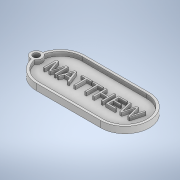
# Autodesk Inventor part: name_tag
Saved by Autodesk Inventor 2020 (Build 240168000, 168)
## iProperties
Created: 2022-11-14
Part Number: name_tag
Material: Generic
Document SubType Name: Modeling
Designer: Matthew Ng
Density: 1 g/cm^3
Appearance: Default
Author: Matthew Ng
Autodesk Inventor part; units mm, degrees
ref_plane "YZ Plane" through (0, 0, 0) normal (1, 0, 0) x (0, 1, 0)
ref_plane "XZ Plane" through (0, 0, 0) normal (0, 1, 0) x (-1, 0, 0)
ref_plane "XY Plane" through (0, 0, 0) normal (0, 0, 1) x (1, 0, 0)
sketch "Sketch1" plane through (0, 0, 0) normal (0, 1, 0) x (-1, 0, 0)
  line L0 (-15, 0) -> (-55, 0)
  line L1 (-55, -30) -> (-15, -30)
  arc A0 (-55, 0) -> (-55, -30) centre (-55, -15) ccw
  line L2 (-15, -1.5) -> (-55, -1.5)
  line L3 (-55, -28.5) -> (-15, -28.5)
  arc A1 (-55, -1.5) -> (-55, -28.5) centre (-55, -15) ccw
  circle A2 centre (0, -15) radius 2
  circle A3 centre (0, -15) radius 3.5
  arc A4 (-15, -28.5) -> (-1.8333, -17.9814) centre (-15, -15) ccw
  arc A5 (-1.8333, -12.0186) -> (-15, -1.5) centre (-15, -15) ccw
  arc A6 (-15, -30) -> (-0.4083, -18.4761) centre (-15, -15) ccw
  arc A7 (-0.4083, -11.5239) -> (-15, 0) centre (-15, -15) ccw
  point P0 (0, 0)
  point P1 (-35, -15)
  dimension "d2" = 30
  dimension "d4" = 27
  dimension "d8" = 7
  dimension "d9" = 4
  constraints: 16 point on circle, 8 centre point, 8 end point, 4 tangent, 2 parallel, 1 coincident, 1 horizontal
  measures "d2" distance between parallel lines of L0 L1
  measures "d4" diameter of A1
  measures "d8" diameter of A3
  measures "d9" diameter of A2
extrude "Extrusion1" add sketch "Sketch1" along normal blind 1.5 contours A3 A4 L3 A1 L2 A5
extrude "Extrusion2" add sketch "Sketch1" along normal blind 4 contours A7 A3 A5 L2 A1 L3 A4 A6 L1 A0 L0 | A3
sketch "Sketch2" plane through (0, 1.5, 0) normal (0, 1, 0) x (1, 0, 0)
  line L0 (7.3671, 19.168) -> (39.5227, 19.168) construction
  line L1 (39.5227, 19.168) -> (39.5227, 12.4254) construction
  line L2 (39.5227, 12.4254) -> (7.3671, 12.4254) construction
  line L3 (7.3671, 12.4254) -> (7.3671, 19.168) construction
  line L4 (8.1964, 11.168) -> (8.1964, 19.168)
  line L5 (8.1964, 19.168) -> (9.7878, 19.168)
  line L6 (9.7878, 19.168) -> (11.6842, 13.5034)
  spline S0 degree 2 poles (11.6842, 13.5034) (11.9464, 12.7107) (12.0683, 12.3204) knots 0 0 0 1 1 1
  spline S1 degree 2 poles (12.0683, 12.3204) (12.2025, 12.7534) (12.4951, 13.6009) knots 0 0 0 1 1 1
  line L7 (12.4951, 13.6009) -> (14.4159, 19.168)
  line L8 (14.4159, 19.168) -> (15.8366, 19.168)
  line L9 (15.8366, 19.168) -> (15.8366, 11.168)
  line L10 (15.8366, 11.168) -> (14.8183, 11.168)
  line L11 (14.8183, 11.168) -> (14.8183, 17.8631)
  line L12 (14.8183, 17.8631) -> (12.4829, 11.168)
  line L13 (12.4829, 11.168) -> (11.5317, 11.168)
  line L14 (11.5317, 11.168) -> (9.2147, 17.979)
  line L15 (9.2147, 17.979) -> (9.2147, 11.168)
  line L16 (9.2147, 11.168) -> (8.1964, 11.168)
  line L17 (16.6659, 11.168) -> (19.739, 19.168)
  line L18 (19.739, 19.168) -> (20.8854, 19.168)
  line L19 (20.8854, 19.168) -> (24.1537, 11.168)
  line L20 (24.1537, 11.168) -> (22.9464, 11.168)
  line L21 (22.9464, 11.168) -> (22.0195, 13.5887)
  line L22 (22.0195, 13.5887) -> (18.6659, 13.5887)
  line L23 (18.6659, 13.5887) -> (17.7878, 11.168)
  line L24 (17.7878, 11.168) -> (16.6659, 11.168)
  line L25 (18.9708, 14.4485) -> (21.6903, 14.4485)
  line L26 (21.6903, 14.4485) -> (20.8488, 16.668)
  spline S2 degree 2 poles (20.8488, 16.668) (20.4708, 17.6802) (20.2878, 18.3265) knots 0 0 0 1 1 1
  spline S3 degree 2 poles (20.2878, 18.3265) (20.1293, 17.5582) (19.8549, 16.796) knots 0 0 0 1 1 1
  line L27 (19.8549, 16.796) -> (18.9708, 14.4485)
  line L28 (27.0317, 11.168) -> (27.0317, 18.2229)
  line L29 (27.0317, 18.2229) -> (24.3976, 18.2229)
  line L30 (24.3976, 18.2229) -> (24.3976, 19.168)
  line L31 (24.3976, 19.168) -> (30.739, 19.168)
  line L32 (30.739, 19.168) -> (30.739, 18.2229)
  line L33 (30.739, 18.2229) -> (28.0927, 18.2229)
  line L34 (28.0927, 18.2229) -> (28.0927, 11.168)
  line L35 (28.0927, 11.168) -> (27.0317, 11.168)
  line L36 (33.861, 11.168) -> (33.861, 18.2229)
  line L37 (33.861, 18.2229) -> (31.2269, 18.2229)
  line L38 (31.2269, 18.2229) -> (31.2269, 19.168)
  line L39 (31.2269, 19.168) -> (37.5683, 19.168)
  line L40 (37.5683, 19.168) -> (37.5683, 18.2229)
  line L41 (37.5683, 18.2229) -> (34.922, 18.2229)
  line L42 (34.922, 18.2229) -> (34.922, 11.168)
  line L43 (34.922, 11.168) -> (33.861, 11.168)
  line L44 (38.6964, 11.168) -> (38.6964, 19.168)
  line L45 (38.6964, 19.168) -> (39.7573, 19.168)
  line L46 (39.7573, 19.168) -> (39.7573, 15.8814)
  line L47 (39.7573, 15.8814) -> (43.9037, 15.8814)
  line L48 (43.9037, 15.8814) -> (43.9037, 19.168)
  line L49 (43.9037, 19.168) -> (44.9647, 19.168)
  line L50 (44.9647, 19.168) -> (44.9647, 11.168)
  line L51 (44.9647, 11.168) -> (43.9037, 11.168)
  line L52 (43.9037, 11.168) -> (43.9037, 14.9363)
  line L53 (43.9037, 14.9363) -> (39.7573, 14.9363)
  line L54 (39.7573, 14.9363) -> (39.7573, 11.168)
  line L55 (39.7573, 11.168) -> (38.6964, 11.168)
  line L56 (46.7512, 11.168) -> (46.7512, 19.168)
  line L57 (46.7512, 19.168) -> (52.5439, 19.168)
  line L58 (52.5439, 19.168) -> (52.5439, 18.2229)
  line L59 (52.5439, 18.2229) -> (47.8122, 18.2229)
  line L60 (47.8122, 18.2229) -> (47.8122, 15.7778)
  line L61 (47.8122, 15.7778) -> (52.2451, 15.7778)
  line L62 (52.2451, 15.7778) -> (52.2451, 14.8326)
  line L63 (52.2451, 14.8326) -> (47.8122, 14.8326)
  line L64 (47.8122, 14.8326) -> (47.8122, 12.1131)
  line L65 (47.8122, 12.1131) -> (52.7269, 12.1131)
  line L66 (52.7269, 12.1131) -> (52.7269, 11.168)
  line L67 (52.7269, 11.168) -> (46.7512, 11.168)
  line L68 (55.5805, 11.168) -> (53.4586, 19.168)
  line L69 (53.4586, 19.168) -> (54.5439, 19.168)
  line L70 (54.5439, 19.168) -> (55.7634, 13.9241)
  spline S4 degree 2 poles (55.7634, 13.9241) (55.9586, 13.1009) (56.1049, 12.2839) knots 0 0 0 1 1 1
  spline S5 degree 2 poles (56.1049, 12.2839) (56.4098, 13.5704) (56.4647, 13.7656) knots 0 0 0 1 1 1
  line L71 (56.4647, 13.7656) -> (57.9829, 19.168)
  line L72 (57.9829, 19.168) -> (59.2634, 19.168)
  line L73 (59.2634, 19.168) -> (60.4098, 15.1192)
  spline S6 degree 2 poles (60.4098, 15.1192) (60.8305, 13.6131) (61.0317, 12.2839) knots 0 0 0 1 1 1
  spline S7 degree 2 poles (61.0317, 12.2839) (61.1842, 13.046) (61.4281, 14.0278) knots 0 0 0 1 1 1
  line L74 (61.4281, 14.0278) -> (62.6781, 19.168)
  line L75 (62.6781, 19.168) -> (63.7451, 19.168)
  line L76 (63.7451, 19.168) -> (61.5622, 11.168)
  line L77 (61.5622, 11.168) -> (60.5256, 11.168)
  line L78 (60.5256, 11.168) -> (58.8549, 17.2656)
  spline S8 degree 2 poles (58.8549, 17.2656) (58.6354, 18.0278) (58.5988, 18.2046) knots 0 0 0 1 1 1
  spline S9 degree 2 poles (58.5988, 18.2046) (58.4647, 17.6558) (58.361, 17.2656) knots 0 0 0 1 1 1
  line L79 (58.361, 17.2656) -> (56.672, 11.168)
  line L80 (56.672, 11.168) -> (55.5805, 11.168)
  point P0 (0, 0)
  constraints: 2 other
emboss "Emboss1" sketch "Sketch2" operation add depth 2 direction (0, -1, 0)
body "Solid1"
